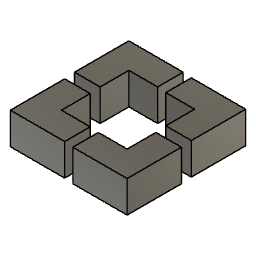
clips (Autodesk Fusion 360 design; units mm, degrees)
Autodesk Fusion 360 part; units mm, degrees
sketch "Esquisse1" plane through (0, 0, 0) normal (0, 0, 1) x (1, 0, 0)
  line L0 (0, 0) -> (0, 10)
  line L1 (0, 10) -> (10, 10)
  line L2 (10, 10) -> (10, 5)
  line L3 (10, 5) -> (5, 5)
  line L4 (5, 5) -> (5, 0)
  line L5 (5, 0) -> (0, 0)
  line L6 (0.28, 0.28) -> (0.28, 9.72)
  line L7 (0.28, 9.72) -> (9.72, 9.72)
  line L8 (9.72, 9.72) -> (9.72, 5.28)
  line L9 (9.72, 5.28) -> (4.72, 5.28)
  line L10 (4.72, 5.28) -> (4.72, 0.28)
  line L11 (4.72, 0.28) -> (0.28, 0.28)
  dimension "d1" = 0.28
  constraint coincident L0.start L5.end
  constraint vertical L0
  constraint perpendicular L0 L1
  constraint perpendicular L1 L2
  constraint perpendicular L2 L3
  constraint perpendicular L3 L4
  constraint perpendicular L0 L5
extrude "Extrusion1" add sketch "Esquisse1" along normal blind 5.5 contours L6 L7 L8 L9 L10 L11 makes body 1
copy_body "Copier/Coller des corps1" bodies 1 makes body 2
move_body "Déplacer1" bodies 2 to x (0, -1, 0) y (1, 0, 0) z (0, 0, 1) at (14, 9.56, 0)
move_body "Déplacer2" bodies 2 to x (1, 0, 0) y (0, 1, 0) z (0, 0, 1) at (-3, 0.3, 0)
copy_body "Copier/Coller des corps2" bodies 2 1 makes body 3 makes body 4
move_body "Déplacer3" bodies 3 4 to x (-1, 0, 0) y (0, -1, 0) z (0, 0, 1) at (21.14, -1.44, 0)
